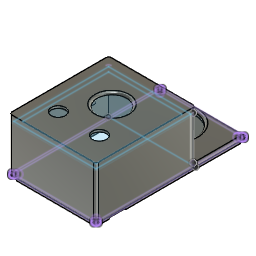
boxv3 top v27 (Autodesk Fusion 360 design; units mm, degrees)
part number: Document
Autodesk Fusion 360 part; units mm, degrees
note: some values were not read from the file. Chosen so that the rebuilt part matches the saved one: that a step has no effect; which pieces of a blend or face edit are solid. Set by a fixed rule: which sketch regions a step uses.
sketch "rpi holes" plane through (0, 0, 0) normal (0, 0, 1) x (1, 0, 0)
  circle A0 centre (-29.0023, 13.5106) radius 1.3509 construction
  circle A1 centre (28.992, 13.5105) radius 1.3509 construction
  circle A2 centre (29.0074, -9.499) radius 1.3509 construction
  circle A3 centre (-28.9869, -9.4988) radius 1.3509 construction
  line L0 (-29.0023, 13.5106) -> (-28.9869, -9.4988) construction
  line L1 (-28.9869, -9.4988) -> (29.0074, -9.499) construction
  line L2 (29.0074, -9.499) -> (28.992, 13.5105) construction
  line L3 (28.992, 13.5105) -> (-29.0023, 13.5106) construction
  constraint coincident A0.centre L0.start
  constraint coincident A3.centre L0.end
  constraint coincident A2.centre L1.end
  constraint coincident A1.centre L2.end
  constraint parallel L1 L3
  constraint parallel L0 L2
  constraint equal L1 L3
  constraint equal A1 A2
  constraint equal A0 A1
  constraint equal A0 A3
sketch "Sketch2" plane through (0, 0, 0) normal (0, 0, 1) x (1, 0, 0)
  line L0 (-32.5, 15) -> (32.5, 15) construction
  line L1 (32.5, 15) -> (32.5, -15) construction
  line L2 (32.5, -15) -> (-32.5, -15) construction
  line L3 (-32.5, -15) -> (-32.5, 15) construction
  line L4 (32.5, 15) -> (37.5, 15) construction
  line L5 (37.5, 15) -> (37.5, -15) construction
  line L6 (37.5, -15) -> (32.5, -15) construction
  line L7 (32.5, -15) -> (32.5, 15) construction
  dimension "d4" = 65
  dimension "d5" = 30
  dimension "d6" = 5
  constraint horizontal L0
  constraint perpendicular L0 L1
  constraint parallel L0 L2
  constraint parallel L1 L3
  constraint horizontal L4
  constraint vertical L5
  constraint horizontal L6
  constraint vertical L7
  measures "d4" distance of L1.end L2.end
  measures "d5" distance of L0.end L1.end
  measures "d6" distance of L0.end L4.end
sketch "Sketch3" plane through (0, 0, 0) normal (0, 0, 1) x (1, 0, 0)
  line L0 (-35, 18) -> (-35, -18)
  line L1 (-35, -18) -> (37, -18)
  line L2 (37, -18) -> (41, -18)
  line L3 (41, -18) -> (41, 18)
  line L4 (41, 18) -> (41, 114)
  line L5 (41, 114) -> (-35, 114)
  line L6 (-35, 114) -> (-35, 18)
  dimension "d37" = 35
  dimension "d40" = 41
  dimension "d41" = 132
  dimension "d42" = 18
  constraint horizontal L2
  constraint vertical L3
  constraint vertical L4
  constraint horizontal L5
  constraint vertical L6
  measures "d37" distance of origin L0
  measures "d40" distance of L3 origin
  measures "d41" distance of L1 L5
  measures "d42" distance of L1 origin
extrude "Extrude1" add sketch "Sketch3" against normal blind 2 makes body 1
sketch "Sketch4" plane through (0, 0, 0) normal (0, 0, 1) x (1, 0, 0)
  circle A0 centre (-29, 13.5) radius 3.25
  circle A1 centre (29, 13.5) radius 3.25
  circle A2 centre (-29, -9.5) radius 3.25
  circle A3 centre (29, -9.5) radius 3.25
  line L0 (-29, 13.5) -> (-29, -9.5) construction
  line L1 (-29, -9.5) -> (29, -9.5) construction
  line L2 (29, -9.5) -> (29, 13.5) construction
  line L3 (29, 13.5) -> (-29, 13.5) construction
  dimension "d12" = 6.5
  dimension "d13" = 6.5
  dimension "d14" = 6.5
  dimension "d15" = 6.5
  constraint coincident A0.centre L0.start
  constraint coincident A2.centre L0.end
  constraint vertical L0
  constraint coincident A3.centre L1.end
  constraint perpendicular L0 L1
  constraint coincident A1.centre L2.end
  constraint perpendicular L1 L2
  constraint perpendicular L0 L3
  measures "d12" diameter of A0
  measures "d13" diameter of A1
  measures "d14" diameter of A2
  measures "d15" diameter of A3
extrude "Extrude2" add sketch "Sketch4" along normal blind 4 bodies 1
sketch "Sketch6" plane through (0, 0, 4) normal (0, 0, 1) x (-1, 0, 0)
  circle A0 centre (29, 9.5) radius 3.25
  point P0 (29.0023, -13.5106)
  point P1 (28.9869, 9.4988)
  point P2 (-29.0074, 9.499)
  point P3 (-28.992, -13.5105)
hole "Hole1" at (-29.0023, 13.5106, 4) at (-28.9869, -9.4988, 4) at (29.0074, -9.499, 4) at (28.992, 13.5105, 4) direction (0, 0, -1) diameter 3.3 depth 4 tip angle 180 bodies 1
sketch "Sketch7" plane through (0, 0, 0) normal (0, 0, 1) x (-1, 0, 0)
  line L0 (35, -114) -> (35, 18)
  line L1 (35, 18) -> (-41, 18)
  line L2 (-41, 18) -> (-41, -114)
  line L3 (35, -114) -> (-41, -114)
  line L4 (-41, -114) -> (-41, 18)
  line L5 (-41, 18) -> (35, 18)
  line L6 (35, 18) -> (35, -114)
  line L7 (-39, 16) -> (33, 16)
  line L8 (33, 16) -> (33, -112)
  line L9 (33, -112) -> (-39, -112)
  line L10 (-39, -112) -> (-39, 16)
  line L11 (-41, -114) -> (35, -114)
  circle A0 centre (-29, 9.5) radius 3.25
  circle A1 centre (29, -13.5) radius 3.25
  circle A2 centre (-29, -13.5) radius 3.25
  circle A3 centre (29, 9.5) radius 3.25
  dimension "d21" = 2
  constraint horizontal L3
  constraint vertical L4
  constraint horizontal L5
  constraint vertical L6
  constraint coincident L1.end L2.start
  constraint coincident L0.start L3.start
extrude "Extrude3" add sketch "Sketch7" along normal blind 14 contours L0 L1 L2 L3 L4 L5 L6 L11 bodies 1
fillet "Fillet1" radius 2 4 edges at (41, -18, 6) (41, 114, 6) (-35, -18, 6) (-35, 114, 6) on bodies 1
fillet "Fillet3" radius 2 4 edges at (-33, 112, 7) (-33, -16, 7) (39, 112, 7) (39, -16, 7) on bodies 1
sketch "Sketch8" plane through (41, 0, 0) normal (1, 0, 0) x (0, 1, 0)
  line L0 (112, -2) -> (112, 14)
  line L1 (112, 14) -> (-16, 14)
  line L2 (-16, 14) -> (-16, -2)
  line L3 (-16, -2) -> (112, -2)
  line L4 (10, 4) -> (-4, 4)
  line L5 (-4, 4) -> (-4, 11)
  line L6 (-4, 11) -> (10, 11)
  line L7 (10, 11) -> (10, 4)
  dimension "d34" = 14
  dimension "d35" = 4
  dimension "d38" = 6
  dimension "d39" = 7
  constraint horizontal L4
  constraint vertical L5
  constraint horizontal L6
  constraint vertical L7
  measures "d34" distance of L5 L7
  measures "d35" horizontal distance of origin L4.end
  measures "d38" distance of L3 L4
  measures "d39" distance of L4 L6
extrude "Extrude4" cut sketch "Sketch8" against normal blind 79 contours L4 L5 L6 L7 bodies 1
chamfer "Smusso1" distance 2 angle 45 4 edges at (25.9699, 14.6753, 0) (-32.0301, 14.6753, 0) (-32.0301, -8.3248, 0) (25.9699, -8.3248, 0) on bodies 1
sketch "Schizzo9" plane through (0, 0, 0) normal (0, 0, 1) x (1, 0, 0)
  line L0 (-20.533, 106.0819) -> (20.467, 106.0819) construction
  line L1 (20.467, 106.0819) -> (20.467, 35.0819) construction
  line L2 (20.467, 35.0819) -> (-20.533, 35.0819) construction
  line L3 (-20.533, 35.0819) -> (-20.533, 106.0819) construction
  line L4 (-20.533, 106.0819) -> (20.467, 35.0819) construction
  line L5 (20.467, 106.0819) -> (-20.533, 35.0819) construction
  circle A0 centre (-20.533, 106.0819) radius 3.25
  circle A1 centre (-20.533, 35.0819) radius 3.25
  circle A2 centre (20.467, 106.0819) radius 3.25
  circle A3 centre (20.467, 35.0819) radius 3.25
  point P0 (-0.033, 70.5819)
  dimension "d43" = 41
  dimension "d44" = 71
  dimension "d45" = 6.5
  constraint horizontal L0
  constraint perpendicular L0 L1
  constraint parallel L0 L2
  constraint parallel L1 L3
  constraint coincident L4 P0
  constraint coincident L5 P0
  constraint coincident L0.start L3.end
  constraint coincident L2.end L3.start
  constraint coincident L0.end L1.start
  constraint coincident L1.end L2.start
  constraint equal A0 A2
  constraint equal A0 A3
  constraint equal A0 A1
  measures "d43" distance of L1.end L2.end
  measures "d44" distance of L0.end L1.end
  measures "d45" diameter of A0
extrude "Estrusione5" add sketch "Schizzo9" along normal blind 8 bodies 1
chamfer "Smusso2" distance 2 angle 45 4 edges at (-23.5631, 36.2571, 0) (17.4369, 36.2571, 0) (17.4369, 107.2571, 0) (-23.5631, 107.2571, 0) on bodies 1
sketch "Schizzo10" plane through (0, 0, 8) normal (0, 0, 1) x (-1, 0, 0)
  circle A0 centre (20.533, -106.0819) radius 3.25
  point P0 (20.533, -106.0819)
  point P1 (-20.467, -106.0819)
  point P2 (-20.467, -35.0819)
  point P3 (20.533, -35.0819)
hole "Foratura2" at (-20.533, 106.0819, 8) at (20.467, 106.0819, 8) at (20.467, 35.0819, 8) at (-20.533, 35.0819, 8) direction (0, 0, -1) diameter 3.4 depth 4 tip angle 118 bodies 1
sketch "Schizzo11" plane through (0, 0, 14) normal (0, 0, 1) x (-1, 0, 0) in component "Component"
  line L0 (31, -112) -> (-37, -112)
  arc A0 (-39, -110) -> (-37, -112) centre (-37, -110) ccw
  line L1 (-39, -110) -> (-39, 14)
  arc A1 (-37, 16) -> (-39, 14) centre (-37, 14) ccw
  line L2 (-37, 16) -> (31, 16)
  arc A2 (33, 14) -> (31, 16) centre (31, 14) ccw
  line L3 (33, 14) -> (33, -110)
  arc A3 (31, -112) -> (33, -110) centre (31, -110) ccw
  arc A4 (33, -114) -> (35, -112) centre (33, -112) ccw
  line L4 (35, -112) -> (35, 16)
  arc A5 (35, 16) -> (33, 18) centre (33, 16) ccw
  line L5 (33, 18) -> (-39, 18)
  arc A6 (-39, 18) -> (-41, 16) centre (-39, 16) ccw
  line L6 (-41, 16) -> (-41, -112)
  arc A7 (-41, -112) -> (-39, -114) centre (-39, -112) ccw
  line L7 (-39, -114) -> (33, -114)
  line L8 (35, -69) -> (-41, -69)
  dimension "d53" = 45
  constraint coincident L4 L8.start
  constraint coincident L6 L8.end
  constraint perpendicular L6 L8
  measures "d53" distance of L7 L8
extrude "Estrusione1" add sketch "Schizzo11" along normal blind 2 separate body contours L0 A0 L1 L3 A3 A4 L4 L6 A7 L7 L8 | L0 A0 L1 L3 A3 L8 makes body 2 in component "Component"
sketch "Schizzo1" plane through (0, 0, 16) normal (0, 0, 1) x (-1, 0, 0) in component "Component"
  line L0 (35, -69) -> (-41, -69)
  line L1 (-41, -69) -> (-41, -112)
  arc A0 (-41, -112) -> (-39, -114) centre (-39, -112) ccw
  line L2 (-39, -114) -> (33, -114)
  arc A1 (33, -114) -> (35, -112) centre (33, -112) ccw
  line L3 (35, -112) -> (35, -69)
  circle A2 centre (0, -90.5) radius 21
  dimension "d67" = 42
  dimension "d68" = 23.5
  dimension "d69" = 35
  measures "d67" diameter of A2
  measures "d68" distance of L2 A2.centre
  measures "d69" distance of L3 A2.centre
extrude "Estrusione4" add sketch "Schizzo1" against normal blind 6 contours A2 bodies 2 in component "Component"
hole "Foratura1" at (0, 90.5, 16) direction (0, 0, -1) diameter 39 depth 4 tip angle 180 bodies 2 in component "Component"
sketch "Schizzo2" plane through (0, 0, 14) normal (0, 0, 1) x (-1, 0, 0) in component "Component"
  line L0 (31, -112) -> (-37, -112)
  arc A0 (-39, -110) -> (-37, -112) centre (-37, -110) ccw
  line L1 (-39, -110) -> (-39, 14)
  arc A1 (-37, 16) -> (-39, 14) centre (-37, 14) ccw
  line L2 (-37, 16) -> (31, 16)
  arc A2 (33, 14) -> (31, 16) centre (31, 14) ccw
  line L3 (33, 14) -> (33, -110)
  arc A3 (31, -112) -> (33, -110) centre (31, -110) ccw
  arc A4 (33, -114) -> (35, -112) centre (33, -112) ccw
  line L4 (35, -112) -> (35, 16)
  arc A5 (35, 16) -> (33, 18) centre (33, 16) ccw
  line L5 (33, 18) -> (-39, 18)
  arc A6 (-39, 18) -> (-41, 16) centre (-39, 16) ccw
  line L6 (-41, 16) -> (-41, -112)
  arc A7 (-41, -112) -> (-39, -114) centre (-39, -112) ccw
  line L7 (-39, -114) -> (33, -114)
  line L8 (35, -69) -> (-41, -69)
  constraint coincident L4 L8.start
  constraint coincident L6 L8.end
  constraint perpendicular L6 L8
extrude "Estrusione5'" add sketch "Schizzo2" along normal blind 40 contours L1 A1 L2 A2 L3 L4 A5 L5 A6 L6 L8 bodies 2 in component "Component"
sketch "Schizzo3" plane through (39, 0, 0) normal (-1, 0, 0) x (0, -1, 0) in component "Component"
  line L0 (-69, 14) -> (14, 14)
  line L1 (14, 14) -> (14, 54)
  line L2 (14, 54) -> (-69, 54)
  line L3 (-69, 54) -> (-69, 16)
  line L4 (-69, 16) -> (-69, 14)
  line L5 (-69, 54) -> (-67, 54)
  line L6 (-67, 54) -> (-67, 16)
  line L7 (-67, 16) -> (-69, 16)
  line L8 (-69, 16) -> (-69, 54)
  point P0 (-69, 16)
  dimension "d77" = 2
  constraint horizontal L5
  constraint vertical L6
  constraint horizontal L7
  constraint vertical L8
  constraint coincident L2.end L3.start
  constraint coincident P0 L3.end
  measures "d77" distance of L2.end L5.end
extrude "Estrusione6" add sketch "Schizzo3" along normal blind 74 contours L2 L3 L5 L6 L7 L8 bodies 2 in component "Component"
fillet "Raccordo1" radius 2 2 edges at (41, 69, 35) (-35, 69, 35) on bodies 2 in component "Component"
sketch "Schizzo5" plane through (0, 0, 54) normal (0, 0, 1) x (-1, 0, 0) in component "Component"
  line L0 (35, -67) -> (35, 16)
  arc A0 (35, 16) -> (33, 18) centre (33, 16) ccw
  line L1 (33, 18) -> (-39, 18)
  arc A1 (-39, 18) -> (-41, 16) centre (-39, 16) ccw
  line L2 (-41, 16) -> (-41, -67)
  line L3 (-39, -69) -> (33, -69)
  line L4 (33, -67) -> (-39, -67)
  line L5 (-39, -67) -> (-39, 14)
  arc A2 (-37, 16) -> (-39, 14) centre (-37, 14) ccw
  line L6 (-37, 16) -> (31, 16)
  arc A3 (33, 14) -> (31, 16) centre (31, 14) ccw
  line L7 (33, 14) -> (33, -67)
  arc A4 (33, -69) -> (35, -67) centre (33, -67) ccw
  arc A5 (-41, -67) -> (-39, -69) centre (-39, -67) ccw
extrude "Estrusione8" add sketch "Schizzo5" along normal blind 6 contours L0 A0 L1 A1 L2 L3 A4 A5 | L4 L5 A2 L6 A3 L7 bodies 2 in component "Component"
fillet "Raccordo3" [suppressed] in component "Component"
sketch "Schizzo6" plane through (0, 0, 54) normal (0, 0, -1) x (1, 0, 0) in component "Component"
  line L0 (-33, -67) -> (39, -67)
  line L1 (39, -67) -> (39, 14)
  arc A0 (39, 14) -> (37, 16) centre (37, 14) ccw
  line L2 (37, 16) -> (-31, 16)
  arc A1 (-31, 16) -> (-33, 14) centre (-31, 14) ccw
  line L3 (-33, 14) -> (-33, -67)
sketch "Schizzo8" plane through (0, 0, 54) normal (0, 0, -1) x (1, 0, 0) in component "Component"
  line L0 (39, -67) -> (-33, -67)
  line L1 (-33, -67) -> (-33, 16)
  line L2 (-33, 16) -> (39, 16)
  line L3 (39, 16) -> (39, -67)
  line L4 (-29, 12) -> (35, 12)
  line L5 (35, 12) -> (35, -63)
  line L6 (35, -63) -> (-29, -63)
  line L7 (-29, -63) -> (-29, 12)
  dimension "d104" = 4
  constraint horizontal L0
  constraint vertical L1
  constraint horizontal L2
  constraint vertical L3
extrude "Estrusione12" cut sketch "Schizzo8" against normal blind 4 contours L4 L5 L6 L7 bodies 2 in component "Component"
fillet "Raccordo4" radius 2 4 edges at (3, 63, 54) (35, 25.5, 54) (3, -12, 54) (-29, 25.5, 54) on bodies 2 in component "Component"
fillet "Raccordo5" radius 2 4 edges at (3, 63, 58) (35, 25.5, 58) (-29, 25.5, 58) (3, -12, 58) on bodies 2 in component "Component"
extrude "Estrusione13" add 1 faces at (-9, 68.3333, 16) along direction (0, 0, -1) blind 2 on bodies 2 bodies 2 in component "Component"
sketch "Schizzo10 (2)" plane through (0, 0, 60) normal (0, 0, 1) x (-1, 0, 0) in component "Component"
  circle A0 centre (-3, -34) radius 13
  circle A1 centre (15.5, -34) radius 3
  circle A2 centre (-21.5, -34) radius 3
  line L0 (15.5, -34) -> (-3, -34) construction
  line L1 (-3, -34) -> (-21.5, -34) construction
  line L2 (15.5, -34) -> (25, -34) construction
  line L3 (-21.5, -34) -> (-31, -34) construction
  line L4 (-3, -34) -> (-3, 8) construction
  line L5 (-3, -34) -> (-3, -59) construction
  line L6 (-39, -69) -> (33, -69)
  line L7 (35, -67) -> (35, 16)
  arc A3 (35, 16) -> (33, 18) centre (33, 16) ccw
  line L8 (33, 18) -> (-39, 18)
  arc A4 (-39, 18) -> (-41, 16) centre (-39, 16) ccw
  line L9 (-41, 16) -> (-41, -67)
  arc A5 (-41, -67) -> (-39, -69) centre (-39, -67) ccw
  arc A6 (33, -69) -> (35, -67) centre (33, -67) ccw
  line L10 (-3, -59) -> (-3, -69) construction
  circle A7 centre (-21, -5) radius 6.25
  circle A8 centre (15, -5) radius 6.25
  line L11 (-21, -5) -> (-41, -5) construction
  line L12 (-21, -5) -> (15, -5) construction
  line L13 (15, -5) -> (35, -5) construction
  dimension "d113" = 26
  dimension "d114" = 6
  dimension "d115" = 6
  dimension "d116" = 18.5
  dimension "d153" = 25
  dimension "d154" = 10
  dimension "d155" = 12.5
  constraint coincident A1.centre L0.start
  constraint coincident A0.centre L0.end
  constraint horizontal L0
  constraint coincident A2.centre L1.end
  constraint horizontal L1
  constraint equal L0 L1
  constraint equal L2 L3
  constraint midpoint L6 L10.end
  constraint perpendicular L6 L10
  constraint equal A7 A8
  constraint coincident A7.centre L11.start
  constraint coincident L9 L11.end
  constraint perpendicular L9 L11
  constraint coincident A8.centre L12.end
  constraint parallel L11 L12
  constraint coincident L7 L13.end
  constraint perpendicular L7 L13
  constraint equal L11 L13
  measures "d113" diameter of A0
  measures "d114" diameter of A1
  measures "d115" diameter of A2
  measures "d116" distance of A0.centre A1.centre
  measures "d153" distance of A0.centre L5.end
  measures "d154" distance of L5.end L10.end
  measures "d155" diameter of A7
extrude "Estrusione14" add sketch "Schizzo10 (2)" against normal blind 8 contours A1 | A2 bodies 2 in component "Component"
extrude "Estrusione15" cut sketch "Schizzo10 (2)" against normal blind 2 contours A0 bodies 2 in component "Component"
chamfer "Smusso2'" distance 2 angle 45 2 edges at (24.297, 35.0848, 58) (-12.703, 35.0848, 58) on bodies 2 in component "Component"
sketch "Schizzo11 (2)" plane through (0, 0, 52) normal (0, 0, -1) x (1, 0, 0) in component "Component"
  circle A0 centre (21.5, -34) radius 3
  point P0 (21.5, -34)
  point P1 (-15.5, -34)
hole "Foratura3" at (21.5, 34, 52) at (-15.5, 34, 52) direction (0, 0, 1) diameter 3.4 depth 6 tip angle 180 bodies 2 in component "Component"
sketch "Schizzo17" plane through (0, 0, 14) normal (0, 0, -1) x (1, 0, 0) in component "Component"
  line L0 (-33, -67) -> (-33, 14)
  arc A0 (-31, 16) -> (-33, 14) centre (-31, 14) ccw
  line L1 (-31, 16) -> (37, 16)
  arc A1 (39, 14) -> (37, 16) centre (37, 14) ccw
  line L2 (39, 14) -> (39, -67)
  line L3 (39, -67) -> (-33, -67)
  line L4 (41, -112) -> (41, 16)
  arc A2 (41, 16) -> (39, 18) centre (39, 16) ccw
  line L5 (39, 18) -> (-33, 18)
  arc A3 (-33, 18) -> (-35, 16) centre (-33, 16) ccw
  line L6 (-35, 16) -> (-35, -112)
  circle A4 centre (0, -90.5) radius 21
  arc A5 (-35, -112) -> (-33, -114) centre (-33, -112) ccw
  line L7 (-33, -114) -> (39, -114)
  arc A6 (39, -114) -> (41, -112) centre (39, -112) ccw
  line L8 (-31.3, -67) -> (-31.3, 14)
  arc A7 (-31, 14.3) -> (-31.3, 14) centre (-31, 14) ccw
  line L9 (-31, 14.3) -> (37, 14.3)
  arc A8 (37.3, 14) -> (37, 14.3) centre (37, 14) ccw
  line L10 (37.3, 14) -> (37.3, -67)
  dimension "d133" = 1.7
extrude "Estrusione18" add sketch "Schizzo17" against normal blind 4 contours L0 A0 L1 A1 L2 L3 L8 A7 L9 A8 L10 bodies 2 in component "Component"
fillet "Raccordo6" radius 2 3 edges at (37.3, 26.5, 18) (3, -14.3, 18) (-31.3, 26.5, 18) on bodies 2 in component "Component"
sketch "Schizzo18" plane through (0, 0, 14) normal (0, 0, -1) x (1, 0, 0) in component "Component"
  line L0 (37.3, -67) -> (-31.3, -67)
  line L1 (-31.3, -67) -> (-31.3, 14)
  line L2 (-31, 14.3) -> (37, 14.3)
  line L3 (37.3, 14) -> (37.3, -67)
  line L4 (41, -112) -> (41, 16)
  arc A0 (41, 16) -> (39, 18) centre (39, 16) ccw
  line L5 (39, 18) -> (-33, 18)
  arc A1 (-33, 18) -> (-35, 16) centre (-33, 16) ccw
  line L6 (-35, 16) -> (-35, -112)
  circle A2 centre (0, -90.5) radius 21
  line L7 (-32.8, -65) -> (-32.8, 13.8)
  line L8 (-30.8, 15.8) -> (36.8, 15.8)
  line L9 (38.8, 13.8) -> (38.8, -65)
  line L10 (-30.8, -67) -> (-31.3, -67)
  line L11 (36.8, -67) -> (37.3, -67)
  arc A3 (-35, -112) -> (-33, -114) centre (-33, -112) ccw
  line L12 (-33, -114) -> (39, -114)
  arc A4 (39, -114) -> (41, -112) centre (39, -112) ccw
  arc A5 (-30.8, 15.8) -> (-32.8, 13.8) centre (-30.8, 13.8) ccw
  arc A6 (38.8, 13.8) -> (36.8, 15.8) centre (36.8, 13.8) ccw
  line L13 (-32.8, -65) -> (-32.8, -110)
  line L14 (38.8, -65) -> (38.9915, -109.9915)
  line L15 (36.9915, -112) -> (-30.8, -112)
  line L16 (-31.3, -67) -> (-31.3, -110.0004)
  line L17 (37.3, -67) -> (37.3, -110.0004)
  line L18 (37.3, -110.0004) -> (-31.3, -110.0004)
  arc A7 (36.9915, -112) -> (38.9915, -109.9915) centre (36.9915, -110) ccw
  arc A8 (-32.8, -110) -> (-30.8, -112) centre (-30.8, -110) ccw
  arc A9 (-31, 14.3) -> (-31.3, 14) centre (-31, 14) ccw
  arc A10 (37.3, 14) -> (37, 14.3) centre (37, 14) ccw
  dimension "d144" = 2
  dimension "d145" = 2
  dimension "d146" = 2
  constraint coincident L0.end L1.start
  constraint perpendicular L7 L10
  constraint coincident L0.start L3.end
  constraint perpendicular L3 L11
  constraint tangent L7 A5
  constraint tangent L8 A5
  constraint tangent L8 A6
  constraint tangent L9 A6
  constraint equal A5 A6
  constraint parallel L7 L13
  constraint perpendicular L10 L16
  constraint perpendicular L0 L17
  constraint perpendicular L16 L18
  constraint tangent L14 A7
  constraint tangent L15 A7
  constraint tangent L15 A8
  constraint tangent L13 A8
  measures "d144" radius of A5
  measures "d145" radius of A7
  measures "d146" radius of A8
extrude "Estrusione19" add sketch "Schizzo18" along normal blind 4 contours L7 L8 L9 A5 A6 L13 L14 L15 A7 A8 bodies 2 in component "Component"
fillet "Raccordo2" [no effect] in component "Component"
sketch "Schizzo19" plane through (0, 0, 12) normal (0, 0, 1) x (-1, 0, 0) in component "Component"
  line L0 (46.5905, -125.2541) -> (-50.6418, -125.2541)
  line L1 (-50.6418, -125.2541) -> (-50.6418, -68.8054)
  line L2 (-50.6418, -68.8054) -> (46.5905, -68.8054)
  line L3 (46.5905, -68.8054) -> (46.5905, -125.2541)
  constraint horizontal L0
  constraint vertical L1
  constraint horizontal L2
  constraint vertical L3
extrude "Estrusione20" [suppressed] in component "Component"
fillet "Raccordo7" radius 2 1 edges at (15.1203, 29.299, 60) on bodies 2 in component "Component"
fillet "Raccordo8" radius 2 1 edges at (-18.1804, 97.5515, 16) on bodies 2 in component "Component"
sketch "Schizzo20" plane through (41, 0, 0) normal (1, 0, 0) x (0, 1, 0) in component "Component"
  line L0 (-4, 4) -> (-4, 11)
  line L1 (-4, 11) -> (10, 11)
  line L2 (10, 11) -> (10, 4)
  line L3 (10, 4) -> (-4, 4)
  line L4 (112, -2) -> (112, 14)
  line L5 (112, 14) -> (-16, 14)
  line L6 (-16, 14) -> (-16, -2)
  line L7 (-16, -2) -> (112, -2)
extrude "Estrusione21" cut sketch "Schizzo20" against normal blind 95 contours L0 L1 L2 L3 bodies 2 in component "Component"
extrude "Estrusione22" cut sketch "Schizzo10 (2)" against normal blind 3 contours A7 | A8 bodies 2 in component "Component"
fillet "Raccordo9" radius 2 5 edges at (41, 89.5, 16) (40.4142, 113.4142, 16) (3, 114, 16) (-34.4142, 113.4142, 16) (-35, 89.5, 16) on bodies 2 in component "Component"
fillet "Raccordo4'" radius 1 8 edges at (40, 10, 11) (40, -4, 11) (40, 10, 4) (40, -4, 4) (-34, -4, 4) (-34, 10, 4) (-34, 10, 11) (-34, -4, 11) on bodies 1
component "Component" placed x (1, 0, 0) y (0, 1, 0) z (0, 0, 1) at (0, 0, 0)
